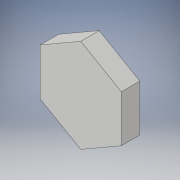
# Autodesk Inventor part: Half Hexagon Test v1
Saved by Autodesk Inventor 2019 (Build 230136000, 136)
## iProperties
Created: 2021-08-21
Part Number: Half Hexagon Test v1
Material: Generic
Document SubType Name: Modeling
Designer: Lix
Density: 1 g/cm^3
Appearance: Default
Author: Lix
Autodesk Inventor part; units mm, degrees
ref_plane "YZ Plane" through (0, 0, 0) normal (1, 0, 0) x (0, 1, 0)
ref_plane "XZ Plane" through (0, 0, 0) normal (0, 1, 0) x (-1, 0, 0)
ref_plane "XY Plane" through (0, 0, 0) normal (0, 0, 1) x (1, 0, 0)
sketch "Sketch2" plane through (0, 0, 0) normal (0, 0, 1) x (1, 0, 0)
  line L0 (0, -101.0363) -> (-87.5, -50.5181)
  line L1 (-87.5, -50.5181) -> (-87.5, 50.5181)
  line L2 (-87.5, 50.5181) -> (0, 101.0363)
  line L3 (0, 101.0363) -> (87.5, 50.5181)
  line L4 (87.5, 50.5181) -> (87.5, -50.5181)
  line L5 (87.5, -50.5181) -> (0, -101.0363)
  point P0 (0, 0)
  point P1 (0, 0)
  dimension "d4" = 175
  constraints: 12 end point, 1 coincident, 1 vertical, 13 other
  measures "d4" distance between parallel lines of L0 L3
extrude "Extrusion2" add sketch "Sketch2" along normal blind 40
body "Solid2"
